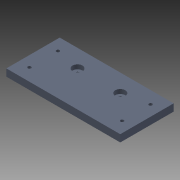
# Autodesk Inventor part: 1_0204_012
Saved by Autodesk Inventor 2012 SP1 (Build 160190100, 190)
## iProperties
Created: 2013-03-27
Part Number: 1_0204_012
Material: Default
Document SubType Name: Modeling
Designer: vogel
Density: 1 g/cm^3
Author: vogel
Autodesk Inventor part; units mm, degrees
ref_plane "YZ Plane" through (0, 0, 0) normal (1, 0, 0) x (0, 1, 0)
ref_plane "XZ Plane" through (0, 0, 0) normal (0, 1, 0) x (-1, 0, 0)
ref_plane "XY Plane" through (0, 0, 0) normal (0, 0, 1) x (1, 0, 0)
sketch "Skizze1" plane through (0, 0, 0) normal (0, 0, 1) x (1, 0, 0)
  line L0 (-80, 25) -> (80, 25)
  line L1 (80, 25) -> (80, -50)
  line L2 (80, -50) -> (-80, -50)
  line L3 (-80, -50) -> (-80, 25)
  line L4 (-112, 0) -> (112, 0) projected
  line L5 (0, -65) -> (0, 40) projected
  circle A0 centre (-30, 0) radius 2.7
  circle A1 centre (30, 0) radius 2.7
  point P0 (0, 0)
  dimension "d0" = 25
  dimension "d1" = 160
  dimension "d2" = 60
  dimension "d3" = 5.4
  dimension "d4" = 75
  constraints: 8 end point, 2 centre point, 2 coincident, 2 parallel, 2 point on line, 1 equal radius, 1 horizontal, 1 perpendicular, 1 symmetric about line, 1 other
  measures "d0" distance between parallel lines of L0 L4
  measures "d1" distance of L0.start L0.end
  measures "d2" distance of point (30, 0) point (-30, 0)
  measures "d3" diameter of A0
  measures "d4" distance of L2.end L0.start
extrude "Extrusion1" add sketch "Skizze1" along normal blind 10 contours L0 L5 L4 A0 L3 | L0 L1 L4 A1 L5 | L4 A0 L5 L2 L3 | L4 A1 L1 L2 L5
sketch "Skizze3" plane through (0, 0, 10) normal (0, 0, 1) x (1, 0, 0)
  circle A0 centre (30, 0) radius 2.7 projected
  circle A1 centre (-30, 0) radius 2.7 projected
  circle A2 centre (-30, 0) radius 7
  circle A3 centre (30, 0) radius 7
  point P0 (0, 0)
  dimension "d8" = 14
  constraints: 2 centre point, 2 coincident, 1 equal radius
  measures "d8" diameter of A2
extrude "Extrusion2" cut sketch "Skizze3" against normal blind 6
sketch "Skizze4" plane through (0, 0, 0) normal (0, 0, -1) x (-1, 0, 0)
  line L0 (80, 25) -> (-80, 25) projected
  line L1 (-80, 25) -> (-80, -50) projected
  line L2 (-80, -50) -> (80, -50) projected
  line L3 (80, -50) -> (80, 25) projected
  line L4 (0, -50) -> (0, 25)
  line L5 (-65, -50) -> (-65, 25)
  line L6 (65, -50) -> (65, 25)
  line L7 (-80, -12.5) -> (80, -12.5)
  point P0 (0, 0)
  point P1 (-65, 7.5)
  point P2 (-65, -32.5)
  point P3 (65, -32.5)
  point P4 (65, 7.5)
  dimension "d11" = 130
  dimension "d12" = 40
  constraints: 8 end point, 8 point on line, 4 midpoint, 2 horizontal alignment, 2 perpendicular, 1 symmetric about line, 1 other
  measures "d11" distance between parallel lines of L6 L5
  measures "d12" distance of point (-65, -32.5) point (-65, 7.5)
hole "Bohrung1" at (65, 7.5, 0) at (65, -32.5, 0) at (-65, -32.5, 0) at (-65, 7.5, 0) direction (0, 0, 1) diameter 4.5 end through all counterbore diameter 8 counterbore depth 6
